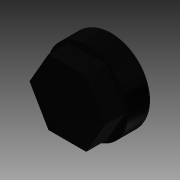
# Autodesk Inventor part: servo_nut_2_for_FatShark_180MG
Saved by Autodesk Inventor 2015 SP1 (Build 190203100, 203)
## iProperties
Created: 2015-07-16
Part Number: servo_nut_2_for_FatShark_180MG
Material: Generic
Document SubType Name: Modeling
Designer: Alexandre Cherpillod
Density: 1 g/cm^3
Appearance: Smooth - Black
Mass: 0.197532 g
Surface Area: 2.02891 cm^2
Volume: 0.197532 cm^3
Author: Alexandre Cherpillod
Autodesk Inventor part; units mm, degrees
ref_plane "YZ Plane" through (0, 0, 0) normal (1, 0, 0) x (0, 1, 0)
ref_plane "XZ Plane" through (0, 0, 0) normal (0, 1, 0) x (-1, 0, 0)
ref_plane "XY Plane" through (0, 0, 0) normal (0, 0, 1) x (1, 0, 0)
sketch "Sketch1" plane through (0, 0, 0) normal (0, 1, 0) x (-1, 0, 0)
  line L0 (3.7528, 0) -> (1.8764, -3.25)
  line L1 (1.8764, -3.25) -> (-1.8764, -3.25)
  line L2 (-1.8764, -3.25) -> (-3.7528, 0)
  line L3 (-3.7528, 0) -> (-1.8764, 3.25)
  line L4 (-1.8764, 3.25) -> (1.8764, 3.25)
  line L5 (1.8764, 3.25) -> (3.7528, 0)
  point P0 (0, 0)
  point P1 (0, 0)
  dimension "d0" = 6.5
  constraints: 12 end point, 1 coincident, 13 other
  measures "d0" distance between parallel lines of L2 L5
extrude "Extrusion1" add sketch "Sketch1" along normal blind 2
sketch "Sketch2" plane through (0, 2, 0) normal (0, 1, 0) x (1, 0, 0)
  circle A0 centre (0, 0) radius 4
  dimension "d3" = 8
  constraints: 1 centre point, 1 coincident
  measures "d3" diameter of A0
extrude "Extrusion2" add sketch "Sketch2" along normal blind 2.5
fillet "Fillet1" radius 0.5 1 edges at (-4, 4.5, 0)
body "Solid1"
